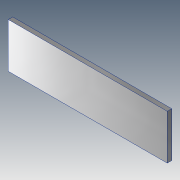
# Autodesk Inventor part: Frame bottom Left
Saved by Autodesk Inventor 2019 (Build 230136000, 136)
## iProperties
Created: 2018-10-20
Part Number: Frame bottom Left
Material: Aluminum 6061
Document SubType Name: Modeling
Designer: LillaHunden
Density: 2.7 g/cm^3
Appearance: Aluminum - Flat
Mass: 172.125 g
Surface Area: 285.5 cm^2
Volume: 63.75 cm^3
Author: LillaHunden
Autodesk Inventor part; units mm, degrees
ref_plane "YZ Plane" through (0, 0, 0) normal (1, 0, 0) x (0, 1, 0)
ref_plane "XZ Plane" through (0, 0, 0) normal (0, 1, 0) x (-1, 0, 0)
ref_plane "XY Plane" through (0, 0, 0) normal (0, 0, 1) x (1, 0, 0)
sketch "Sketch1" plane through (0, 0, 0) normal (0, 0, 1) x (1, 0, 0)
  line L0 (169.989, 31) -> (-92.011, 31) projected
  line L1 (169.989, 31) -> (169.989, 40.9823) projected
  line L2 (-92.011, 40.9823) -> (169.989, 40.9823) projected
  line L3 (-92.011, 31) -> (-92.011, 40.9823) projected
  line L4 (-102.011, 50.9479) -> (179.989, 50.9479)
  line L5 (179.989, 50.9479) -> (179.989, 0.9479)
  line L6 (179.989, 0.9479) -> (-102.011, 0.9479)
  line L7 (-102.011, 0.9479) -> (-102.011, 50.9479)
  dimension "d4" = 50
  dimension "d5" = 10
  dimension "d6" = 10
  constraints: 8 end point, 2 parallel, 1 horizontal, 1 perpendicular
  measures "d4" distance of L4.end L5.end
  measures "d5" distance between parallel lines of L5 L1
  measures "d6" distance between parallel lines of L7 L3
extrude "Extrusion1" add sketch "Sketch1" along normal blind 10 contours L0 L3 L2 L1 | L4 L5 L6 L7
body "Solid1"
